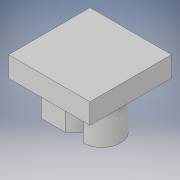
# Autodesk Inventor part: 5
Saved by Autodesk Inventor 2019 (Build 230136000, 136)
## iProperties
Created: 2018-08-09
Part Number: 5
Material: Generic
Document SubType Name: Modeling
Designer: Ge Shi
Density: 1 g/cm^3
Appearance: Default
Author: Ge Shi
Autodesk Inventor part; units mm, degrees
ref_plane "YZ Plane" through (0, 0, 0) normal (1, 0, 0) x (0, 1, 0)
ref_plane "XZ Plane" through (0, 0, 0) normal (0, 1, 0) x (-1, 0, 0)
ref_plane "XY Plane" through (0, 0, 0) normal (0, 0, 1) x (1, 0, 0)
sketch "Sketch1" plane through (0, 0, 0) normal (0, 1, 0) x (-1, 0, 0)
  line L0 (-10, -10) -> (10, -10)
  line L1 (10, -10) -> (10, 10)
  line L2 (10, 10) -> (-10, 10)
  line L3 (-10, 10) -> (-10, -10)
  line L4 (-10, -10) -> (10, 10) construction
  line L5 (10, -10) -> (-10, 10) construction
  line L6 (7.5, 4.5) -> (7.5, -4.5)
  line L7 (7.5, -4.5) -> (5, -4.5)
  line L8 (5, -4.5) -> (5, 2)
  line L9 (7.5, 4.5) -> (1.5711, 4.5)
  arc A0 (-2.9289, 2.0711) -> (-1.4645, 1.4645) centre (-2.9289, 0) ccw
  line L10 (1.5711, 4.5) -> (-1.4645, 1.4645)
  line L11 (-7.5, 0) -> (-7.5, -3.5066) construction
  line L12 (14, 0) -> (-14, 0) projected
  arc A1 (-2.9289, 4.5711) -> (1.5448, 0.9382) centre (-2.9289, 0) ccw
  line L13 (-2.9289, 4.5711) -> (-2.9289, 2.0711)
  line L14 (1.5448, 0.9382) -> (2.6066, 2)
  line L15 (2.6066, 2) -> (5, 2)
  point P0 (0, 0)
  dimension "d0" = 20
  dimension "d1" = 20
  dimension "d2" = 2.5
  dimension "d3" = 2.5
  dimension "d4" = 2.5
  dimension "d8" = 2.5
  dimension "d9" = 9
  dimension "d10" = 2.5
  dimension "d11" = 2.5
  constraints: 30 end point, 4 parallel, 4 point on circle, 3 horizontal, 3 perpendicular, 3 point on line, 3 vertical, 2 centre point, 2 midpoint, 1 coincident, 1 line through centre, 1 tangent, 1 other
  measures "d0" distance of L2.end L1.end
  measures "d1" distance of L0.end L1.end
  measures "d2" distance of L6.end L7.end
  measures "d3" distance between parallel lines of L3 L11
  measures "d4" distance between parallel lines of L1 L6
  measures "d8" radial gap between concentric circles of A0 A1
  measures "d9" distance of L6.start L6.end
  measures "d10" distance between parallel lines of L9 L15
  measures "d11" distance between parallel lines of L10 L14
extrude "Extrusion1" add sketch "Sketch1" against normal blind 10 contours A1 L13 A0 L12 | L12 A0 A1 | L12 L8 L15 L14 A1 A0 L10 L9 L6 | L6 L7 L8 L12
extrude "Extrusion2" add sketch "Sketch1" along normal blind 5
body "Solid1"
